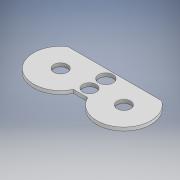
# Autodesk Inventor part: paitent remote top
Saved by Autodesk Inventor 2021 (Build 250183000, 183)
## iProperties
Created: 2023-01-12
Part Number: paitent remote top
Material: Generic
Document SubType Name: Modeling
Designer: boyle
Density: 1 g/cm^3
Appearance: Default
Author: boyle
Autodesk Inventor part; units mm, degrees
ref_plane "YZ Plane" through (0, 0, 0) normal (1, 0, 0) x (0, 1, 0)
ref_plane "XZ Plane" through (0, 0, 0) normal (0, 1, 0) x (-1, 0, 0)
ref_plane "XY Plane" through (0, 0, 0) normal (0, 0, 1) x (1, 0, 0)
sketch "Sketch1" plane through (0, 0, 0) normal (0, 1, 0) x (-1, 0, 0)
  line L0 (-23.3466, 0) -> (-154.4106, 0)
  line L1 (-98.9962, 48.2251) -> (-78.8108, 48.2251)
  line L2 (-88.9, 0) -> (-23.3466, 0)
  line L3 (-88.9, 0) -> (-154.4106, 0)
  arc A0 (-98.9962, 48.2251) -> (-154.4106, 0) centre (-133.35, 31.75) ccw
  arc A1 (-23.3466, 0) -> (-78.8108, 48.2251) centre (-44.4805, 31.7012) ccw
  point P0 (0, 0)
  dimension "d0" = 76.2
  dimension "d1" = 76.2
  dimension "d2" = 131.064
  constraints: 8 end point, 4 point on circle, 2 centre point, 2 collinear, 1 horizontal, 1 parallel, 1 point on line
  measures "d0" diameter of A0
  measures "d1" diameter of A1
  measures "d2" distance of L0.start L0.end
extrude "Extrusion1" add sketch "Sketch1" along normal blind 4.826
sketch "Sketch2" plane through (0, 4.826, 0) normal (0, 1, 0) x (1, 0, 0)
  line L0 (154.4106, 0) -> (23.3466, 0) projected
  arc A0 (23.3466, 0) -> (78.8108, -48.2251) centre (44.4805, -31.7012) ccw projected
  line L1 (78.8108, -48.2251) -> (98.9962, -48.2251) projected
  arc A1 (98.9962, -48.2251) -> (154.4106, 0) centre (133.35, -31.75) ccw projected
  circle A2 centre (44.4805, -31.7012) radius 9.525
  circle A3 centre (133.35, -31.75) radius 9.525
  line L2 (88.8786, 0) -> (88.9035, -48.2251)
  circle A4 centre (88.891, -35.624) radius 9.525
  line L3 (88.891, -24.1125) -> (88.8786, 0)
  circle A5 centre (88.8826, -12.5545) radius 10.16
  point P0 (0, 0)
  dimension "d5" = 19.05
  dimension "d6" = 20.32
  constraints: 4 centre point, 4 end point, 2 coincident, 2 equal radius, 2 midpoint
  measures "d5" diameter of A4
  measures "d6" diameter of A5
extrude "Extrusion2" cut sketch "Sketch2" against normal through all contours A5 L2 | L2 A5 | A4 L2 | L2 A4 | A2 | A3
body "Solid1"
